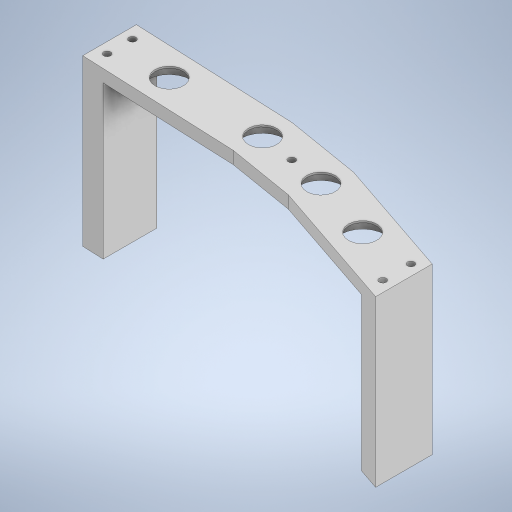
# Autodesk Inventor part: Servo Holder
Saved by Autodesk Inventor 2023 (Build 270158000, 158)
## iProperties
Created: 2022-10-14
Part Number: Servo Holder
Material: Generic
Document SubType Name: Modeling
Designer: GROS
Density: 1 g/cm^3
Appearance: Default
Author: GROS
Autodesk Inventor part; units mm, degrees
ref_plane "YZ Plane" through (0, 0, 0) normal (1, 0, 0) x (0, 1, 0)
ref_plane "XZ Plane" through (0, 0, 0) normal (0, 1, 0) x (-1, 0, 0)
ref_plane "XY Plane" through (0, 0, 0) normal (0, 0, 1) x (1, 0, 0)
sketch "Sketch1" plane through (0, 0, 0) normal (0, 1, 0) x (-1, 0, 0)
  circle A0 centre (92.6541, -28.2127) radius 6.05
  circle A1 centre (65.1803, -27.0368) radius 6.05
  circle A2 centre (45.4573, -23.7633) radius 6.05
  circle A3 centre (92.6541, -28.2127) radius 7.55
  circle A4 centre (65.1803, -27.0368) radius 7.55
  circle A5 centre (45.4573, -23.7633) radius 7.55
  circle A6 centre (92.6541, -28.2127) radius 4
  circle A7 centre (45.4573, -23.7633) radius 4
  line L0 (92.6541, -28.2127) -> (100.2041, -28.2127)
  line L1 (70.678, -35.6025) -> (39.5208, -30.4313)
  line L2 (60.2143, -34.3811) -> (122.676, -37.0546)
  line L3 (51.451, -33.7618) -> (1.5927, -16.8916)
  line L4 (51.8932, -17.9704) -> (4.2209, -1.8399)
  circle A8 centre (27.7249, -17.7633) radius 4
  circle A9 centre (27.7249, -17.7633) radius 6.05
  circle A10 centre (27.7249, -17.7633) radius 7.55
  line L5 (27.7249, -17.7633) -> (20.1749, -17.7633)
  line L6 (20.1749, -17.7633) -> (16.1749, -17.7633)
  line L7 (16.1749, -17.7633) -> (10.1749, -17.7633)
  line L8 (10.1749, -17.7633) -> (10.1749, -19.7955)
  line L9 (10.1749, -19.7955) -> (10.1749, -3.8545)
  line L10 (13.1749, -17.7633) -> (13.1749, -20.8106)
  line L11 (13.1749, -20.8106) -> (13.1749, -4.8696)
  line L12 (13.1749, -20.8106) -> (13.1749, -16.8106)
  line L13 (13.1749, -4.8696) -> (13.1749, -8.8696)
  circle A11 centre (13.1749, -16.8106) radius 1
  circle A12 centre (13.1749, -8.8696) radius 1
  line L14 (16.1749, -17.7633) -> (16.1749, -21.8257)
  line L15 (16.1749, -17.7633) -> (16.1749, -5.8847)
  line L16 (114.6217, -21.596) -> (60.8612, -19.295)
  line L17 (100.2041, -28.2127) -> (104.2041, -28.2127)
  line L18 (104.2041, -28.2127) -> (110.2041, -28.2127)
  line L19 (107.2041, -28.2127) -> (107.2041, -21.2785)
  line L20 (107.2041, -28.2127) -> (107.2041, -36.3923)
  line L21 (107.2041, -36.3923) -> (107.2041, -28.3923)
  line L22 (107.2041, -21.2785) -> (107.2041, -25.2785)
  circle A13 centre (107.2041, -32.3923) radius 1
  circle A14 centre (107.2041, -25.2785) radius 1
  line L23 (110.2041, -28.2127) -> (110.2041, -36.5208)
  line L24 (104.2041, -28.2127) -> (104.2041, -36.2639)
  line L25 (104.2041, -28.2127) -> (104.2041, -21.1501)
  line L26 (110.2041, -28.2127) -> (110.2041, -21.4069)
  line L27 (75.2254, -21.0507) -> (39.3363, -15.0941)
  line L28 (65.1803, -27.0368) -> (45.4573, -27.0368)
  line L29 (55.3188, -33.0533) -> (55.3188, -17.7467)
  circle A15 centre (55.3188, -25.4) radius 1
  circle A16 centre (55.3188, -25.4) radius 2.55
  circle A17 centre (65.1803, -27.0368) radius 4
  point P0 (43.6173, -31.1112)
  point P1 (64.3979, -34.5602)
  point P2 (65.9627, -19.5133)
  point P3 (66.4165, -19.5886)
  point P4 (65.5031, -19.4937)
  point P5 (47.2973, -16.4154)
  point P6 (47.8772, -16.6116)
  point P7 (46.6935, -16.3152)
  dimension "d143" = 15.1
  dimension "d132" = 12.1
  dimension "d133" = 12.1
  dimension "d134" = 12.1
  dimension "d135" = 15.1
  dimension "d136" = 15.1
  dimension "d137" = 8
  dimension "d139" = 8
  dimension "d140" = 1.1759
  dimension "d141" = 3.2735
  dimension "d142" = 12.1
  dimension "d144" = 8
  dimension "d145" = 6
  dimension "d146" = 4
  dimension "d147" = 6
  dimension "d148" = 4
  dimension "d149" = 4
  dimension "d150" = 2
  dimension "d151" = 2
  dimension "d152" = 4
  dimension "d153" = 6
  dimension "d154" = 4
  dimension "d155" = 4
  dimension "d156" = 2
  dimension "d157" = 2
  dimension "d159" = 5.1
  dimension "d160" = 2
  dimension "d161" = 8
  constraints: 60 end point, 22 point on line, 16 centre point, 13 coincident, 8 tangent, 5 vertical, 4 horizontal, 4 midpoint, 2 horizontal alignment, 1 parallel, 8 other
  measures "d132" diameter of A0
  measures "d133" diameter of A1
  measures "d134" diameter of A2
  measures "d135" diameter of A4
  measures "d136" diameter of A5
  measures "d137" diameter of A6
  measures "d139" diameter of A7
  measures "d140" vertical distance of A4.centre point (92.654, -28.213)
  measures "d141" vertical distance of A5.centre A4.centre
  measures "d142" diameter of A9
  measures "d144" diameter of A8
  measures "d145" vertical distance of point (27.725, -17.763) A2.centre
  measures "d146" distance of L5.end L7.start
  measures "d147" distance of L7.start L7.end
  measures "d148" distance of L11.end L13.end
  measures "d149" distance of L10.end L12.end
  measures "d150" diameter of A11
  measures "d151" diameter of A12
  measures "d152" distance of L17.start L25.start
  measures "d153" distance of L25.start L26.start
  measures "d154" distance of L19.end L22.end
  measures "d155" distance of point (107.204, -32.392) L20.end
  measures "d156" diameter of A14
  measures "d157" diameter of A13
  measures "d159" diameter of A16
  measures "d160" diameter of A15
  measures "d161" diameter of A17
extrude "Extrusion1" add sketch "Sketch1" against normal blind 3 contours A3 | A3 L16 L25 L17 | L17 L24 L2 A3 | A3 L2 A4 L27 L16 | L27 A4 L16 | L16 A4 A16 L29 L27 | L2 L1 A4 | A4 A16 | L29 A16 A5 L4 L27 | L1 L29 A16 L28 A4 | A16 A4 | A4 A16 L28 L29 A15 | L27 A5 L3 A10 L4 | L4 A5 L27 | L29 A15 L28 A16 A5 | L28 A16 A4 | L1 A5 L28 A16 L29 | A5 A16 | A10 L6 L15 L4 | A10 | A15 L29 | L29 A15 | A5 A16 | A16 L29 L28 | L1 L3 A5 | A16 L28 L29 | A10 L3 L14 L6 | A16 L28 A5
extrude "Extrusion2" add sketch "Sketch1" along normal blind 0.5 contours A0 | A3 | A3 L16 L25 L17 | L17 L24 L2 A3 | A3 L2 A4 L27 L16 | L25 L16 L19 A14 L18 | L18 L20 A13 L2 L24 | L27 A4 L16 | L16 A4 A16 L29 L27 | L2 L1 A4 | A1 | A4 A16 | L19 A14 L16 L26 L18 | L18 L23 L2 L20 A13 | L29 A16 A5 L4 L27 | L1 L29 A16 L28 A4 | A16 A4 | A4 A16 L28 L29 A15 | L27 A5 L3 A10 L4 | L4 A5 L27 | L29 A15 L28 A16 A5 | L28 A16 A4 | L1 A5 L28 A16 L29 | A2 | A5 A16 | A10 L6 L15 L4 | A9 | A10 | A15 L29 | L29 A15 | A5 A16 | A16 L29 L28 | L1 L3 A5 | A16 L28 L29 | L15 L7 A11 L11 A12 L4 | A10 L3 L14 L6 | A16 L28 A5 | L11 A12 A11 L7 L9 L4 | L14 L3 L10 A11 L7 | L7 A11 L10 L3 L8
extrude "Extrusion8" add sketch "Sketch1" against normal blind 46 contours L25 L16 L19 A14 L18 | L18 L20 A13 L2 L24 | L19 A14 L16 L26 L18 | L18 L23 L2 L20 A13 | L15 L7 A11 L11 A12 L4 | L11 A12 A11 L7 L9 L4 | L14 L3 L10 A11 L7 | L7 A11 L10 L3 L8
extrude "Extrusion9" cut sketch "Sketch1" along normal through all both and the other way through all contours A15 L29 | L29 A15
body "Solid1"
